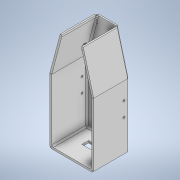
# Autodesk Inventor part: the box
Saved by Autodesk Inventor 2022 (Build 260153000, 153)
## iProperties
Created: 2022-12-16
Part Number: the box
Material: Generic
Document SubType Name: Modeling
Designer: chris
Density: 1 g/cm^3
Appearance: Default
Author: chris
Autodesk Inventor part; units mm, degrees
ref_plane "YZ Plane" through (0, 0, 0) normal (1, 0, 0) x (0, 1, 0)
ref_plane "XZ Plane" through (0, 0, 0) normal (0, 1, 0) x (-1, 0, 0)
ref_plane "XY Plane" through (0, 0, 0) normal (0, 0, 1) x (1, 0, 0)
sketch "Sketch1" plane through (0, 0, 0) normal (0, 0, 1) x (1, 0, 0)
  line L0 (0, 0) -> (80, 0)
  line L1 (80, 0) -> (80, 125.359)
  line L2 (60, 200) -> (80, 125.359)
  line L3 (60, 200) -> (137.2741, 200) construction
  line L4 (0, 0) -> (0, 125.359)
  line L5 (20, 200) -> (0, 125.359)
  line L6 (84, 125.8856) -> (84, -4)
  line L7 (84, -4) -> (-4, -4)
  line L8 (-4, -4) -> (-4, 125.8856)
  line L9 (-4, 125.8856) -> (16.9307, 204)
  line L10 (63.0693, 204) -> (84, 125.8856)
  line L11 (20, 204) -> (20, 200)
  line L12 (60, 200) -> (60, 204)
  line L13 (16.9307, 204) -> (20, 204)
  line L14 (60, 204) -> (63.0693, 204)
  point P0 (40, 0)
  dimension "d0" = 80
  dimension "d4" = 75
  dimension "d5" = 4
  constraints: 30 end point, 4 perpendicular, 2 horizontal, 1 equal length, 1 midpoint, 1 vertical, 3 other
  measures "d0" distance of L0.start L0.end
  measures "d4" angle of L2 L3
  measures "d5" distance between parallel lines of L2 L10
extrude "Extrusion1" add sketch "Sketch1" along normal blind 70
sketch "Sketch2" plane through (0, 0, 0) normal (0, 0, -1) x (-1, 0, 0)
  line L0 (-16.9307, 204) -> (4, 125.8856) projected
  line L1 (-84, 125.8856) -> (-63.0693, 204) projected
  line L2 (-16.9307, 204) -> (-63.0693, 204)
  line L3 (-80, 125.359) -> (-80, 0) projected
  line L4 (-60, 200) -> (-80, 125.359) projected
  line L5 (-60, 204) -> (-60, 200) projected
  line L6 (-63.0693, 204) -> (-60, 204) projected
  line L7 (-84, 125.8856) -> (-63.0693, 204) projected
  line L8 (-84, -4) -> (-84, 125.8856) projected
  line L9 (4, -4) -> (-84, -4) projected
  line L10 (4, 125.8856) -> (4, -4) projected
  line L11 (-16.9307, 204) -> (4, 125.8856) projected
  line L12 (-20, 204) -> (-16.9307, 204) projected
  line L13 (-20, 200) -> (-20, 204) projected
  line L14 (0, 125.359) -> (-20, 200) projected
  line L15 (0, 0) -> (0, 125.359) projected
  line L16 (-80, 0) -> (0, 0) projected
  constraints: 2 end point, 1 horizontal
extrude "Extrusion2" add sketch "Sketch2" along normal blind 3
chamfer "Chamfer1" distance 5 angle 45 5 edges at (40, -4, -3) (84, 60.9428, -3) (-4, 60.9428, -3) (6.4653, 164.9428, -3) (73.5347, 164.9428, -3)
chamfer "Chamfer2" distance 3 angle 45 7 edges at (20, 202, 0) (10, 162.6795, 0) (60, 202, 0) (70, 162.6795, 0) (80, 62.6795, 0) (0, 62.6795, 0) (40, 0, 0)
chamfer "Chamfer3" distance 3 angle 45 4 edges at (84, -4, 36) (-4, -4, 36) (0, 0, 36.5) (80, 0, 36.5)
sketch "Sketch3" plane through (0, 0, 70) normal (0, 0, 1) x (1, 0, 0)
  line L0 (77, 0) -> (78.5, 1.5) projected
  line L1 (81, -4) -> (82.5, -2.5) projected
  line L2 (78.5, 1.5) -> (82.5, -2.5)
  line L3 (79, 1) -> (82.5, -2.5) projected
  circle A0 centre (80.75, -0.75) radius 1
  line L4 (-4, -1) -> (-2.5, -2.5) projected
  line L5 (-2.5, -2.5) -> (1.5, 1.5)
  line L6 (0, 3) -> (3, 0) projected
  line L7 (1, 1) -> (-2.5, -2.5) projected
  circle A1 centre (-0.75, -0.75) radius 1
  line L8 (3, 124.964) -> (0, 125.359) projected
  line L9 (16.9307, 204) -> (-4, 125.8856) projected
  line L10 (80, 125.359) -> (77, 124.964) projected
  line L11 (84, -1) -> (84, 125.8856) projected
  line L12 (1, 125.2273) -> (-4, 125.8856) projected
  circle A2 centre (82, 125.6223) radius 1
  circle A3 centre (-2, 125.6223) radius 1
  point P0 (0, 0)
  dimension "d19" = 2
  dimension "d20" = 2
  dimension "d22" = 2
  dimension "d23" = 2
  constraints: 4 centre point, 4 end point, 3 midpoint, 1 perpendicular, 1 point on line
  measures "d19" diameter of A0
  measures "d20" diameter of A1
  measures "d22" diameter of A2
  measures "d23" diameter of A3
extrude "Extrusion3" cut sketch "Sketch3" against normal blind 5
sketch "Sketch4" plane through (22.1071, 204, -3) normal (0, 1, 0) x (1, 0, 0)
  line L0 (35.7859, 0) -> (40.9622, -5) projected
  line L1 (38.374, -2.5) -> (36.3929, -4.5)
  line L2 (34.8929, -3) -> (37.8929, -6) projected
  circle A0 centre (37.3835, -3.5) radius 1
  line L3 (-21.1071, 0) -> (56.8929, 0) projected
  line L4 (17.8929, 0) -> (17.8929, -26)
  circle A1 centre (-1.5976, -3.5) radius 1
  point P0 (-22.1071, -3)
  dimension "d26" = 2
  constraints: 4 end point, 4 midpoint, 2 centre point, 1 symmetric about line, 1 vertical, 1 other
  measures "d26" diameter of A0
extrude "Extrusion4" cut sketch "Sketch4" against normal blind 15
sketch "Sketch5" plane through (0, 0, 0) normal (0, 0, 1) x (1, 0, 0)
  line L0 (77, 3) -> (3, 3) projected
  line L1 (40, 3) -> (40, 43)
  line L2 (40, 43) -> (40, 113)
  line L3 (40, 78) -> (20, 78)
  line L4 (20, 78) -> (20, 55.5)
  line L5 (20, 55.5) -> (60, 55.5)
  line L6 (60, 55.5) -> (60, 100.5)
  line L7 (60, 100.5) -> (20, 100.5)
  line L8 (20, 100.5) -> (20, 78)
  line L9 (40, 78) -> (70, 78)
  line L10 (70, 78) -> (70, 98)
  circle A0 centre (70, 98) radius 1
  line L11 (70, 78) -> (70, 58)
  circle A1 centre (70, 58) radius 1
  circle A2 centre (10, 98) radius 1
  circle A3 centre (10, 58) radius 1
  line L12 (40, 113) -> (40, 133)
  line L13 (40, 133) -> (63.1521, 133)
  line L14 (63.1521, 133) -> (63.1521, 155.7076)
  circle A4 centre (63.1521, 155.7076) radius 1.5
  circle A5 centre (63.1521, 133) radius 1.5
  circle A6 centre (16.8479, 155.7076) radius 1.5
  circle A7 centre (16.8479, 133) radius 1.5
  point P0 (0, 0)
  dimension "d29" = 40
  dimension "d30" = 70
  dimension "d31" = 20
  dimension "d32" = 22.5
  dimension "d33" = 40
  dimension "d34" = 45
  dimension "d35" = 30
  dimension "d36" = 20
  dimension "d37" = 2
  dimension "d38" = 20
  dimension "d39" = 2
  dimension "d40" = 20
  dimension "d41" = 23.1521
  dimension "d42" = 22.7076
  dimension "d43" = 3
  dimension "d44" = 3
  constraints: 28 end point, 8 centre point, 5 perpendicular, 5 vertical, 4 coincident, 4 symmetric about line, 3 horizontal, 2 midpoint, 1 point on line, 4 other
  measures "d29" distance of L1.start L1.end
  measures "d30" distance of L1.end L2.end
  measures "d31" distance of L3.start L3.end
  measures "d32" distance of L3.end L4.end
  measures "d33" distance of L4.end L5.end
  measures "d34" distance of L5.end L6.end
  measures "d35" distance of L3.start L9.end
  measures "d36" distance of L9.end L10.end
  measures "d37" diameter of A0
  measures "d38" distance of L9.end L11.end
  measures "d39" diameter of A1
  measures "d40" distance of L2.end L12.end
  measures "d41" distance of L12.end L13.end
  measures "d42" distance of L13.end L14.end
  measures "d43" diameter of A4
  measures "d44" diameter of A5
extrude "Extrusion5" cut sketch "Sketch5" against normal blind 40
sketch "Sketch7" plane through (-1, -4, 2) normal (0, -1, 0) x (1, 0, 0)
  line L0 (78, 68) -> (4, 68) projected
  line L1 (41, 68) -> (41, 34)
  line L2 (54.7, 34) -> (27.3, 34)
  line L3 (54.7, 34) -> (54.7, 20.8)
  line L4 (54.7, 20.8) -> (27.3, 20.8)
  line L5 (27.3, 34) -> (27.3, 20.8)
  point P0 (1, -2)
  dimension "d47" = 27.4
  dimension "d48" = 34
  dimension "d49" = 13.2
  constraints: 10 end point, 3 vertical, 2 midpoint, 1 coincident, 1 horizontal, 1 horizontal alignment
  measures "d47" distance of L2.start L2.end
  measures "d48" distance of L1.start L1.end
  measures "d49" distance of L2.start L3.end
extrude "Extrusion6" cut sketch "Sketch7" against normal blind 27.4
sketch "Sketch8" plane through (-4, 125.8856, 2) normal (-0.9659, 0.2588, 0) x (0, 0, 1)
  line L0 (-2, 13.7678) -> (-2, 10.7678) projected
  line L1 (-2, 35.7017) -> (-2, 32.7017) projected
  line L2 (3.9828, 34.5121) -> (3.9828, 12.5782)
  line L3 (3.9828, 23.5451) -> (5.9828, 23.5451)
  line L4 (5.9828, 23.5451) -> (12.9828, 23.5451)
  line L5 (12.9828, 23.5451) -> (12.9828, 30.2951)
  line L6 (12.9828, 30.2951) -> (12.9828, 16.7951)
  line L7 (12.9828, 16.7951) -> (5.9828, 16.7951)
  line L8 (5.9828, 16.7951) -> (5.9828, 29.9848)
  line L9 (5.9828, 29.9848) -> (12.9828, 30.2951)
  point P0 (-2, -120.5609)
  point P1 (12.9828, 30.2951)
  dimension "d52" = 2
  dimension "d53" = 7
  dimension "d54" = 6.75
  dimension "d55" = 13.5
  constraints: 16 end point, 3 perpendicular, 3 point on line, 1 coincident, 1 horizontal, 1 midpoint, 1 vertical
  measures "d52" distance of L3.start L3.end
  measures "d53" distance of L3.end L4.end
  measures "d54" distance of L4.end L5.end
  measures "d55" distance of L5.end L6.end
extrude "Extrusion7" cut sketch "Sketch8" against normal blind 9
chamfer "Chamfer4" distance 1 angle 45 4 edges at (5.7728, 154.6308, 14.9828) (2.2788, 141.5908, 14.9828) (2.2788, 141.5908, 7.9828) (5.6925, 154.331, 7.9828)
sketch "Sketch9" plane through (-4, 125.8856, 2) normal (-1, 0, 0) x (0, 0, 1)
  line L0 (1, -0.5266) -> (1, -122.8856) projected
  line L1 (1, -48.8247) -> (7.6436, -48.8247)
  line L2 (7.6436, -48.8247) -> (7.6436, -34.3247)
  line L3 (7.6436, -34.3247) -> (7.6436, -63.3247)
  circle A0 centre (7.6436, -34.3247) radius 2
  circle A1 centre (7.6436, -63.3247) radius 2
  point P0 (-2, -125.8856)
  dimension "d61" = 14.5
  dimension "d62" = 29
  dimension "d63" = 4
  dimension "d64" = 4
  constraints: 6 end point, 2 centre point, 2 coincident, 2 point on line, 1 horizontal, 1 perpendicular
  measures "d61" distance of L1.end L2.end
  measures "d62" distance of L2.end L3.end
  measures "d63" diameter of A0
  measures "d64" diameter of A1
extrude "Extrusion8" cut sketch "Sketch9" against normal blind 999
equation "\"d45\" = d33"
equation "\"d50\" = d47"
body "Solid1"
